Autodesk Fusion 360 part; units mm, degrees
(part 9 of 11)
  spline S49 degree 5 poles (-5.4732, -19.6968) (-5.4704, -19.6982) (-5.465, -19.7011) (-5.4568, -19.7055) (-5.4459, -19.7113) (-5.4323, -19.7184) (-5.4187, -19.7254) (-5.405, -19.7324) (-5.3914, -19.7394) (-5.3777, -19.7462) (-5.364, -19.753) (-5.3504, -19.7597) (-5.3367, -19.7663) (-5.323, -19.7729) (-5.3093, -19.7793) (-5.2955, -19.7857) (-5.2818, -19.7921) (-5.2681, -19.7983) (-5.2544, -19.8045) (-5.2406, -19.8106) (-5.2269, -19.8166) (-5.2131, -19.8226) (-5.1993, -19.8284) (-5.1855, -19.8342) (-5.1718, -19.8399) (-5.158, -19.8456) (-5.1442, -19.8511) (-5.1304, -19.8566) (-5.1166, -19.862) (-5.1028, -19.8673) (-5.089, -19.8725) (-5.0751, -19.8776) (-5.0613, -19.8827) (-5.0475, -19.8877) (-5.0337, -19.8925) (-5.0198, -19.8973) (-5.006, -19.902) (-4.9921, -19.9067) (-4.9783, -19.9112) (-4.9644, -19.9156) (-4.9506, -19.92) (-4.9367, -19.9242) (-4.9229, -19.9284) (-4.909, -19.9325) (-4.8951, -19.9364) (-4.8813, -19.9403) (-4.8674, -19.9441) (-4.8535, -19.9478) (-4.8397, -19.9514) (-4.8258, -19.9548) (-4.8119, -19.9582) (-4.7981, -19.9615) (-4.7842, -19.9646) (-4.7703, -19.9676) (-4.7565, -19.9705) (-4.7426, -19.9733) (-4.7288, -19.976) (-4.7149, -19.9786) (-4.701, -19.9811) (-4.6872, -19.9835) (-4.6733, -19.9857) (-4.6595, -19.9877) (-4.6457, -19.9895) (-4.6318, -19.9912) (-4.618, -19.9927) (-4.6042, -19.9941) (-4.5904, -19.9954) (-4.5766, -19.9965) (-4.5628, -19.9976) (-4.549, -19.9984) (-4.5353, -19.9988) (-4.5243, -19.9987) (-4.516, -19.9984) (-4.5106, -19.998) (-4.5078, -19.9978) knots -1 -1 -1 -1 -1 -1 -0.98571429 -0.97142857 -0.95714286 -0.94285714 -0.92857143 -0.91428571 -0.9 -0.88571429 -0.87142857 -0.85714286 -0.84285714 -0.82857143 -0.81428571 -0.8 -0.78571429 -0.77142857 -0.75714286 -0.74285714 -0.72857143 -0.71428571 -0.7 -0.68571429 -0.67142857 -0.65714286 -0.64285714 -0.62857143 -0.61428571 -0.6 -0.58571429 -0.57142857 -0.55714286 -0.54285714 -0.52857143 -0.51428571 -0.5 -0.48571429 -0.47142857 -0.45714286 -0.44285714 -0.42857143 -0.41428571 -0.4 -0.38571429 -0.37142857 -0.35714286 -0.34285714 -0.32857143 -0.31428571 -0.3 -0.28571429 -0.27142857 -0.25714286 -0.24285714 -0.22857143 -0.21428571 -0.2 -0.18571429 -0.17142857 -0.15714286 -0.14285714 -0.12857143 -0.11428571 -0.1 -0.08571429 -0.07142857 -0.05714286 -0.04285714 -0.02857143 -0.01428571 0 0 0 0 0 0
  line L57 (-4.5078, -19.9978) -> (-4.4395, -19.9925)
  arc A107 (-4.1719, -20.2115) -> (-4.4395, -19.9925) centre (-4.4201, -20.2417) ccw
  arc A108 (-4.1719, -20.2115) -> (-4.1569, -20.3258) centre (1.6741, -19.5) ccw
  arc A109 (-4.3587, -20.6066) -> (-4.1569, -20.3258) centre (-4.4044, -20.3608) ccw
  line L58 (-4.3587, -20.6066) -> (-4.426, -20.6192)
  spline S50 degree 5 poles (-4.426, -20.6192) (-4.4287, -20.6197) (-4.4341, -20.6207) (-4.4422, -20.6225) (-4.4528, -20.6253) (-4.466, -20.6293) (-4.4791, -20.6336) (-4.4921, -20.6382) (-4.5051, -20.6429) (-4.5181, -20.6477) (-4.5311, -20.6526) (-4.5441, -20.6577) (-4.557, -20.6628) (-4.5699, -20.6682) (-4.5828, -20.6737) (-4.5956, -20.6794) (-4.6083, -20.6853) (-4.6211, -20.6913) (-4.6338, -20.6974) (-4.6465, -20.7036) (-4.6591, -20.7099) (-4.6718, -20.7162) (-4.6844, -20.7228) (-4.697, -20.7294) (-4.7095, -20.7361) (-4.722, -20.743) (-4.7345, -20.7499) (-4.747, -20.757) (-4.7595, -20.7641) (-4.7719, -20.7713) (-4.7843, -20.7787) (-4.7966, -20.7861) (-4.809, -20.7936) (-4.8213, -20.8012) (-4.8335, -20.8089) (-4.8458, -20.8167) (-4.858, -20.8246) (-4.8702, -20.8325) (-4.8824, -20.8406) (-4.8946, -20.8487) (-4.9067, -20.8569) (-4.9188, -20.8652) (-4.9309, -20.8736) (-4.9429, -20.8821) (-4.9549, -20.8906) (-4.9669, -20.8992) (-4.9789, -20.9079) (-4.9908, -20.9167) (-5.0027, -20.9256) (-5.0146, -20.9345) (-5.0265, -20.9435) (-5.0383, -20.9526) (-5.0501, -20.9617) (-5.0619, -20.971) (-5.0737, -20.9803) (-5.0854, -20.9896) (-5.0971, -20.9991) (-5.1088, -21.0086) (-5.1204, -21.0182) (-5.132, -21.0279) (-5.1436, -21.0376) (-5.1552, -21.0474) (-5.1667, -21.0573) (-5.1782, -21.0672) (-5.1897, -21.0773) (-5.2012, -21.0873) (-5.2126, -21.0975) (-5.224, -21.1077) (-5.2353, -21.118) (-5.2467, -21.1283) (-5.258, -21.1388) (-5.267, -21.1471) (-5.2738, -21.1535) (-5.2783, -21.1577) (-5.2805, -21.1598) knots 0 0 0 0 0 0 0.01428571 0.02857143 0.04285714 0.05714286 0.07142857 0.08571429 0.1 0.11428571 0.12857143 0.14285714 0.15714286 0.17142857 0.18571429 0.2 0.21428571 0.22857143 0.24285714 0.25714286 0.27142857 0.28571429 0.3 0.31428571 0.32857143 0.34285714 0.35714286 0.37142857 0.38571429 0.4 0.41428571 0.42857143 0.44285714 0.45714286 0.47142857 0.48571429 0.5 0.51428571 0.52857143 0.54285714 0.55714286 0.57142857 0.58571429 0.6 0.61428571 0.62857143 0.64285714 0.65714286 0.67142857 0.68571429 0.7 0.71428571 0.72857143 0.74285714 0.75714286 0.77142857 0.78571429 0.8 0.81428571 0.82857143 0.84285714 0.85714286 0.87142857 0.88571429 0.9 0.91428571 0.92857143 0.94285714 0.95714286 0.97142857 0.98571429 1 1 1 1 1 1
  arc A110 (-5.2805, -21.1598) -> (-5.1787, -21.5399) centre (1.6741, -19.5) ccw
  spline S51 degree 5 poles (-5.1787, -21.5399) (-5.1757, -21.5406) (-5.1697, -21.542) (-5.1607, -21.5441) (-5.1486, -21.5469) (-5.1336, -21.5502) (-5.1186, -21.5535) (-5.1037, -21.5567) (-5.0887, -21.5599) (-5.0737, -21.563) (-5.0587, -21.566) (-5.0438, -21.5689) (-5.0289, -21.5718) (-5.0139, -21.5745) (-4.999, -21.5773) (-4.9841, -21.5799) (-4.9692, -21.5825) (-4.9543, -21.5849) (-4.9395, -21.5874) (-4.9246, -21.5897) (-4.9098, -21.5919) (-4.8949, -21.5941) (-4.8801, -21.5962) (-4.8653, -21.5983) (-4.8505, -21.6002) (-4.8357, -21.6021) (-4.821, -21.6039) (-4.8062, -21.6056) (-4.7915, -21.6072) (-4.7768, -21.6088) (-4.7621, -21.6102) (-4.7474, -21.6116) (-4.7328, -21.6129) (-4.7181, -21.6141) (-4.7035, -21.6153) (-4.6889, -21.6163) (-4.6743, -21.6173) (-4.6597, -21.6182) (-4.6452, -21.619) (-4.6306, -21.6197) (-4.6161, -21.6203) (-4.6017, -21.6208) (-4.5872, -21.6212) (-4.5728, -21.6216) (-4.5583, -21.6218) (-4.5439, -21.622) (-4.5296, -21.622) (-4.5152, -21.622) (-4.5009, -21.6219) (-4.4866, -21.6217) (-4.4723, -21.6213) (-4.4581, -21.6209) (-4.4439, -21.6203) (-4.4297, -21.6197) (-4.4156, -21.6189) (-4.4015, -21.618) (-4.3874, -21.617) (-4.3733, -21.6159) (-4.3593, -21.6147) (-4.3453, -21.6134) (-4.3314, -21.612) (-4.3175, -21.6103) (-4.3036, -21.6085) (-4.2898, -21.6066) (-4.2761, -21.6044) (-4.2624, -21.6022) (-4.2487, -21.5998) (-4.2351, -21.5974) (-4.2215, -21.5949) (-4.208, -21.5921) (-4.1946, -21.5889) (-4.184, -21.586) (-4.1761, -21.5835) (-4.1709, -21.5818) (-4.1683, -21.5809) knots -1 -1 -1 -1 -1 -1 -0.98571429 -0.97142857 -0.95714286 -0.94285714 -0.92857143 -0.91428571 -0.9 -0.88571429 -0.87142857 -0.85714286 -0.84285714 -0.82857143 -0.81428571 -0.8 -0.78571429 -0.77142857 -0.75714286 -0.74285714 -0.72857143 -0.71428571 -0.7 -0.68571429 -0.67142857 -0.65714286 -0.64285714 -0.62857143 -0.61428571 -0.6 -0.58571429 -0.57142857 -0.55714286 -0.54285714 -0.52857143 -0.51428571 -0.5 -0.48571429 -0.47142857 -0.45714286 -0.44285714 -0.42857143 -0.41428571 -0.4 -0.38571429 -0.37142857 -0.35714286 -0.34285714 -0.32857143 -0.31428571 -0.3 -0.28571429 -0.27142857 -0.25714286 -0.24285714 -0.22857143 -0.21428571 -0.2 -0.18571429 -0.17142857 -0.15714286 -0.14285714 -0.12857143 -0.11428571 -0.1 -0.08571429 -0.07142857 -0.05714286 -0.04285714 -0.02857143 -0.01428571 0 0 0 0 0 0
  line L59 (-4.1683, -21.5809) -> (-4.1038, -21.558)
  arc A111 (-3.7886, -21.7004) -> (-4.1038, -21.558) centre (-4.0205, -21.7938) ccw
  arc A112 (-3.7886, -21.7004) -> (-3.7445, -21.8068) centre (1.6741, -19.5) ccw
  arc A113 (-3.8667, -22.1303) -> (-3.7445, -21.8068) centre (-3.9745, -21.9048) ccw
  line L60 (-3.8667, -22.1303) -> (-3.9285, -22.1599)
  spline S52 degree 5 poles (-3.9285, -22.1599) (-3.931, -22.161) (-3.9359, -22.1635) (-3.9432, -22.1673) (-3.9528, -22.1727) (-3.9645, -22.18) (-3.976, -22.1875) (-3.9874, -22.1953) (-3.9988, -22.2033) (-4.0101, -22.2113) (-4.0214, -22.2194) (-4.0326, -22.2276) (-4.0437, -22.236) (-4.0548, -22.2445) (-4.0658, -22.2531) (-4.0767, -22.262) (-4.0875, -22.2709) (-4.0982, -22.28) (-4.109, -22.2892) (-4.1196, -22.2984) (-4.1302, -22.3078) (-4.1408, -22.3173) (-4.1513, -22.3268) (-4.1617, -22.3365) (-4.1721, -22.3462) (-4.1824, -22.3561) (-4.1927, -22.366) (-4.2029, -22.376) (-4.2131, -22.3862) (-4.2232, -22.3964) (-4.2332, -22.4067) (-4.2433, -22.417) (-4.2532, -22.4275) (-4.2632, -22.438) (-4.273, -22.4486) (-4.2828, -22.4593) (-4.2926, -22.4701) (-4.3023, -22.481) (-4.312, -22.4919) (-4.3217, -22.5029) (-4.3312, -22.5139) (-4.3408, -22.5251) (-4.3503, -22.5363) (-4.3597, -22.5476) (-4.3691, -22.559) (-4.3785, -22.5704) (-4.3878, -22.5819) (-4.397, -22.5935) (-4.4063, -22.6051) (-4.4154, -22.6168) (-4.4246, -22.6286) (-4.4336, -22.6404) (-4.4427, -22.6523) (-4.4517, -22.6643) (-4.4606, -22.6763) (-4.4695, -22.6884) (-4.4784, -22.7005) (-4.4872, -22.7128) (-4.4959, -22.725) (-4.5047, -22.7374) (-4.5133, -22.7498) (-4.522, -22.7623) (-4.5306, -22.7748) (-4.5391, -22.7874) (-4.5476, -22.8) (-4.556, -22.8127) (-4.5645, -22.8255) (-4.5728, -22.8383) (-4.5811, -22.8512) (-4.5894, -22.8641) (-4.5977, -22.8771) (-4.6042, -22.8875) (-4.6091, -22.8954) (-4.6123, -22.9006) (-4.614, -22.9033) knots 0 0 0 0 0 0 0.01428571 0.02857143 0.04285714 0.05714286 0.07142857 0.08571429 0.1 0.11428571 0.12857143 0.14285714 0.15714286 0.17142857 0.18571429 0.2 0.21428571 0.22857143 0.24285714 0.25714286 0.27142857 0.28571429 0.3 0.31428571 0.32857143 0.34285714 0.35714286 0.37142857 0.38571429 0.4 0.41428571 0.42857143 0.44285714 0.45714286 0.47142857 0.48571429 0.5 0.51428571 0.52857143 0.54285714 0.55714286 0.57142857 0.58571429 0.6 0.61428571 0.62857143 0.64285714 0.65714286 0.67142857 0.68571429 0.7 0.71428571 0.72857143 0.74285714 0.75714286 0.77142857 0.78571429 0.8 0.81428571 0.82857143 0.84285714 0.85714286 0.87142857 0.88571429 0.9 0.91428571 0.92857143 0.94285714 0.95714286 0.97142857 0.98571429 1 1 1 1 1 1
  arc A114 (-4.614, -22.9033) -> (-4.4172, -23.244) centre (1.6741, -19.5) ccw
  spline S53 degree 5 poles (-4.4172, -23.244) (-4.4141, -23.2439) (-4.408, -23.2438) (-4.3987, -23.2434) (-4.3864, -23.243) (-4.371, -23.2424) (-4.3557, -23.2417) (-4.3404, -23.2409) (-4.3251, -23.24) (-4.3098, -23.2391) (-4.2946, -23.2382) (-4.2794, -23.2371) (-4.2642, -23.236) (-4.2491, -23.2349) (-4.234, -23.2336) (-4.2189, -23.2323) (-4.2039, -23.2309) (-4.1888, -23.2295) (-4.1739, -23.228) (-4.1589, -23.2264) (-4.144, -23.2247) (-4.1291, -23.223) (-4.1142, -23.2212) (-4.0994, -23.2193) (-4.0846, -23.2173) (-4.0699, -23.2153) (-4.0551, -23.2132) (-4.0405, -23.2111) (-4.0258, -23.2088) (-4.0112, -23.2065) (-3.9966, -23.2041) (-3.9821, -23.2017) (-3.9676, -23.1991) (-3.9531, -23.1965) (-3.9387, -23.1938) (-3.9243, -23.1911) (-3.91, -23.1882) (-3.8957, -23.1853) (-3.8814, -23.1823) (-3.8672, -23.1792) (-3.853, -23.1761) (-3.8389, -23.1728) (-3.8248, -23.1695) (-3.8108, -23.1661) (-3.7968, -23.1626) (-3.7829, -23.159) (-3.769, -23.1554) (-3.7551, -23.1516) (-3.7413, -23.1478) (-3.7276, -23.1439) (-3.7139, -23.1399) (-3.7002, -23.1358) (-3.6866, -23.1315) (-3.6731, -23.1272) (-3.6597, -23.1228) (-3.6463, -23.1183) (-3.6329, -23.1137) (-3.6196, -23.109) (-3.6064, -23.1043) (-3.5932, -23.0994) (-3.5801, -23.0943) (-3.5671, -23.0892) (-3.5542, -23.0838) (-3.5414, -23.0784) (-3.5287, -23.0728) (-3.516, -23.067) (-3.5034, -23.0612) (-3.4909, -23.0554) (-3.4784, -23.0494) (-3.4661, -23.0432) (-3.454, -23.0367) (-3.4445, -23.0311) (-3.4375, -23.0267) (-3.433, -23.0237) (-3.4307, -23.0221) knots -1 -1 -1 -1 -1 -1 -0.98571429 -0.97142857 -0.95714286 -0.94285714 -0.92857143 -0.91428571 -0.9 -0.88571429 -0.87142857 -0.85714286 -0.84285714 -0.82857143 -0.81428571 -0.8 -0.78571429 -0.77142857 -0.75714286 -0.74285714 -0.72857143 -0.71428571 -0.7 -0.68571429 -0.67142857 -0.65714286 -0.64285714 -0.62857143 -0.61428571 -0.6 -0.58571429 -0.57142857 -0.55714286 -0.54285714 -0.52857143 -0.51428571 -0.5 -0.48571429 -0.47142857 -0.45714286 -0.44285714 -0.42857143 -0.41428571 -0.4 -0.38571429 -0.37142857 -0.35714286 -0.34285714 -0.32857143 -0.31428571 -0.3 -0.28571429 -0.27142857 -0.25714286 -0.24285714 -0.22857143 -0.21428571 -0.2 -0.18571429 -0.17142857 -0.15714286 -0.14285714 -0.12857143 -0.11428571 -0.1 -0.08571429 -0.07142857 -0.05714286 -0.04285714 -0.02857143 -0.01428571 0 0 0 0 0 0
  line L61 (-3.4307, -23.0221) -> (-3.3742, -22.9833)
  arc A115 (-3.0329, -23.0392) -> (-3.3742, -22.9833) centre (-3.2328, -23.1895) ccw
  arc A116 (-3.0329, -23.0392) -> (-2.9628, -23.1307) centre (1.6741, -19.5) ccw
  arc A117 (-2.9971, -23.4748) -> (-2.9628, -23.1307) centre (-3.1596, -23.2848) ccw
  line L62 (-2.9971, -23.4748) -> (-3.0492, -23.5193)
  spline S54 degree 5 poles (-3.0492, -23.5193) (-3.0513, -23.5211) (-3.0554, -23.5247) (-3.0615, -23.5303) (-3.0693, -23.538) (-3.0787, -23.548) (-3.0879, -23.5583) (-3.0969, -23.5688) (-3.1058, -23.5794) (-3.1147, -23.5901) (-3.1235, -23.6008) (-3.1322, -23.6117) (-3.1408, -23.6226) (-3.1493, -23.6337) (-3.1576, -23.6449) (-3.1659, -23.6563) (-3.174, -23.6677) (-3.182, -23.6793) (-3.19, -23.6909) (-3.1979, -23.7026) (-3.2057, -23.7144) (-3.2135, -23.7263) (-3.2211, -23.7382) (-3.2287, -23.7502) (-3.2362, -23.7623) (-3.2436, -23.7745) (-3.251, -23.7868) (-3.2583, -23.7991) (-3.2655, -23.8115) (-3.2726, -23.824) (-3.2797, -23.8366) (-3.2866, -23.8492) (-3.2936, -23.8619) (-3.3004, -23.8746) (-3.3072, -23.8874) (-3.3139, -23.9003) (-3.3206, -23.9132) (-3.3272, -23.9262) (-3.3337, -23.9393) (-3.3402, -23.9524) (-3.3466, -23.9656) (-3.3529, -23.9788) (-3.3591, -23.9921) (-3.3653, -24.0054) (-3.3715, -24.0188) (-3.3776, -24.0323) (-3.3836, -24.0458) (-3.3895, -24.0594) (-3.3954, -24.073) (-3.4012, -24.0867) (-3.407, -24.1004) (-3.4127, -24.1142) (-3.4184, -24.128) (-3.424, -24.1419) (-3.4295, -24.1558) (-3.435, -24.1698) (-3.4404, -24.1839) (-3.4457, -24.198) (-3.451, -24.2121) (-3.4562, -24.2263) (-3.4614, -24.2405) (-3.4665, -24.2548) (-3.4716, -24.2691) (-3.4766, -24.2834) (-3.4815, -24.2979) (-3.4864, -24.3123) (-3.4912, -24.3268) (-3.496, -24.3414) (-3.5007, -24.356) (-3.5053, -24.3706) (-3.5099, -24.3853) (-3.5135, -24.3971) (-3.5162, -24.4059) (-3.518, -24.4118) (-3.5189, -24.4148) knots 0 0 0 0 0 0 0.01428571 0.02857143 0.04285714 0.05714286 0.07142857 0.08571429 0.1 0.11428571 0.12857143 0.14285714 0.15714286 0.17142857 0.18571429 0.2 0.21428571 0.22857143 0.24285714 0.25714286 0.27142857 0.28571429 0.3 0.31428571 0.32857143 0.34285714 0.35714286 0.37142857 0.38571429 0.4 0.41428571 0.42857143 0.44285714 0.45714286 0.47142857 0.48571429 0.5 0.51428571 0.52857143 0.54285714 0.55714286 0.57142857 0.58571429 0.6 0.61428571 0.62857143 0.64285714 0.65714286 0.67142857 0.68571429 0.7 0.71428571 0.72857143 0.74285714 0.75714286 0.77142857 0.78571429 0.8 0.81428571 0.82857143 0.84285714 0.85714286 0.87142857 0.88571429 0.9 0.91428571 0.92857143 0.94285714 0.95714286 0.97142857 0.98571429 1 1 1 1 1 1
  arc A118 (-3.5189, -24.4148) -> (-3.2406, -24.693) centre (1.6741, -19.5) ccw
  spline S55 degree 5 poles (-3.2406, -24.693) (-3.2377, -24.6921) (-3.2318, -24.6904) (-3.2229, -24.6877) (-3.2111, -24.684) (-3.1965, -24.6794) (-3.1818, -24.6748) (-3.1672, -24.6701) (-3.1527, -24.6653) (-3.1382, -24.6605) (-3.1237, -24.6556) (-3.1093, -24.6507) (-3.0949, -24.6457) (-3.0806, -24.6406) (-3.0663, -24.6355) (-3.0521, -24.6304) (-3.0379, -24.6251) (-3.0238, -24.6198) (-3.0097, -24.6145) (-2.9957, -24.6091) (-2.9817, -24.6036) (-2.9678, -24.5981) (-2.9539, -24.5925) (-2.9401, -24.5869) (-2.9263, -24.5812) (-2.9125, -24.5754) (-2.8989, -24.5696) (-2.8852, -24.5637) (-2.8717, -24.5577) (-2.8582, -24.5517) (-2.8447, -24.5456) (-2.8313, -24.5395) (-2.8179, -24.5333) (-2.8047, -24.527) (-2.7914, -24.5207) (-2.7782, -24.5143) (-2.7651, -24.5078) (-2.7521, -24.5013) (-2.7391, -24.4947) (-2.7261, -24.4881) (-2.7133, -24.4814) (-2.7005, -24.4746) (-2.6877, -24.4677) (-2.675, -24.4608) (-2.6624, -24.4538) (-2.6499, -24.4467) (-2.6374, -24.4396) (-2.625, -24.4324) (-2.6127, -24.4251) (-2.6004, -24.4178) (-2.5882, -24.4104) (-2.5761, -24.4029) (-2.5641, -24.3953) (-2.5521, -24.3876) (-2.5403, -24.3799) (-2.5285, -24.372) (-2.5168, -24.3641) (-2.5051, -24.3562) (-2.4936, -24.3481) (-2.4821, -24.34) (-2.4708, -24.3318) (-2.4596, -24.3234) (-2.4485, -24.3149) (-2.4375, -24.3063) (-2.4267, -24.2976) (-2.416, -24.2888) (-2.4053, -24.2799) (-2.3947, -24.271) (-2.3842, -24.262) (-2.3739, -24.2529) (-2.3639, -24.2434) (-2.3561, -24.2356) (-2.3506, -24.2295) (-2.3469, -24.2254) (-2.3452, -24.2233) knots -1 -1 -1 -1 -1 -1 -0.98571429 -0.97142857 -0.95714286 -0.94285714 -0.92857143 -0.91428571 -0.9 -0.88571429 -0.87142857 -0.85714286 -0.84285714 -0.82857143 -0.81428571 -0.8 -0.78571429 -0.77142857 -0.75714286 -0.74285714 -0.72857143 -0.71428571 -0.7 -0.68571429 -0.67142857 -0.65714286 -0.64285714 -0.62857143 -0.61428571 -0.6 -0.58571429 -0.57142857 -0.55714286 -0.54285714 -0.52857143 -0.51428571 -0.5 -0.48571429 -0.47142857 -0.45714286 -0.44285714 -0.42857143 -0.41428571 -0.4 -0.38571429 -0.37142857 -0.35714286 -0.34285714 -0.32857143 -0.31428571 -0.3 -0.28571429 -0.27142857 -0.25714286 -0.24285714 -0.22857143 -0.21428571 -0.2 -0.18571429 -0.17142857 -0.15714286 -0.14285714 -0.12857143 -0.11428571 -0.1 -0.08571429 -0.07142857 -0.05714286 -0.04285714 -0.02857143 -0.01428571 0 0 0 0 0 0
  line L63 (-2.3452, -24.2233) -> (-2.3006, -24.1713)
  arc A119 (-1.9565, -24.1369) -> (-2.3006, -24.1713) centre (-2.1106, -24.3338) ccw
  arc A120 (-1.9565, -24.1369) -> (-1.8651, -24.2071) centre (1.6741, -19.5) ccw
  arc A121 (-1.8092, -24.5484) -> (-1.8651, -24.2071) centre (-2.0153, -24.4069) ccw
  line L64 (-1.8092, -24.5484) -> (-1.848, -24.6048)
  spline S56 degree 5 poles (-1.848, -24.6048) (-1.8495, -24.6071) (-1.8526, -24.6117) (-1.857, -24.6186) (-1.8626, -24.6281) (-1.8691, -24.6402) (-1.8753, -24.6525) (-1.8812, -24.665) (-1.8871, -24.6776) (-1.8929, -24.6902) (-1.8986, -24.7028) (-1.9042, -24.7155) (-1.9097, -24.7283) (-1.915, -24.7412) (-1.9202, -24.7542) (-1.9252, -24.7673) (-1.9301, -24.7805) (-1.9349, -24.7937) (-1.9396, -24.807) (-1.9442, -24.8204) (-1.9487, -24.8338) (-1.9531, -24.8473) (-1.9574, -24.8608) (-1.9616, -24.8744) (-1.9657, -24.888) (-1.9697, -24.9017) (-1.9737, -24.9154) (-1.9775, -24.9292) (-1.9812, -24.9431) (-1.9849, -24.957) (-1.9885, -24.9709) (-1.992, -24.9849) (-1.9954, -24.999) (-1.9987, -25.013) (-2.0019, -25.0272) (-2.0051, -25.0413) (-2.0082, -25.0556) (-2.0112, -25.0698) (-2.0141, -25.0841) (-2.0169, -25.0985) (-2.0197, -25.1128) (-2.0224, -25.1273) (-2.025, -25.1417) (-2.0275, -25.1562) (-2.03, -25.1708) (-2.0324, -25.1853) (-2.0347, -25.2) (-2.0369, -25.2146) (-2.0391, -25.2293) (-2.0412, -25.244) (-2.0432, -25.2588) (-2.0452, -25.2735) (-2.047, -25.2884) (-2.0488, -25.3032) (-2.0506, -25.3181) (-2.0522, -25.333) (-2.0538, -25.348) (-2.0553, -25.363) (-2.0568, -25.378) (-2.0582, -25.3931) (-2.0595, -25.4081) (-2.0607, -25.4232) (-2.0619, -25.4384) (-2.063, -25.4536) (-2.064, -25.4688) (-2.065, -25.484) (-2.0659, -25.4992) (-2.0667, -25.5145) (-2.0675, -25.5298) (-2.0682, -25.5452) (-2.0688, -25.5605) (-2.0693, -25.5729) (-2.0696, -25.5821) (-2.0698, -25.5883) (-2.0699, -25.5914) knots 0 0 0 0 0 0 0.01428571 0.02857143 0.04285714 0.05714286 0.07142857 0.08571429 0.1 0.11428571 0.12857143 0.14285714 0.15714286 0.17142857 0.18571429 0.2 0.21428571 0.22857143 0.24285714 0.25714286 0.27142857 0.28571429 0.3 0.31428571 0.32857143 0.34285714 0.35714286 0.37142857 0.38571429 0.4 0.41428571 0.42857143 0.44285714 0.45714286 0.47142857 0.48571429 0.5 0.51428571 0.52857143 0.54285714 0.55714286 0.57142857 0.58571429 0.6 0.61428571 0.62857143 0.64285714 0.65714286 0.67142857 0.68571429 0.7 0.71428571 0.72857143 0.74285714 0.75714286 0.77142857 0.78571429 0.8 0.81428571 0.82857143 0.84285714 0.85714286 0.87142857 0.88571429 0.9 0.91428571 0.92857143 0.94285714 0.95714286 0.97142857 0.98571429 1 1 1 1 1 1
  arc A122 (-2.0699, -25.5914) -> (-1.7291, -25.7881) centre (1.6741, -19.5) ccw
  spline S57 degree 5 poles (-1.7291, -25.7881) (-1.7265, -25.7865) (-1.7212, -25.7832) (-1.7134, -25.7783) (-1.7029, -25.7718) (-1.69, -25.7636) (-1.677, -25.7553) (-1.6641, -25.747) (-1.6513, -25.7386) (-1.6386, -25.7302) (-1.6259, -25.7217) (-1.6132, -25.7132) (-1.6006, -25.7047) (-1.5881, -25.6961) (-1.5756, -25.6875) (-1.5632, -25.6788) (-1.5509, -25.6701) (-1.5386, -25.6613) (-1.5264, -25.6525) (-1.5142, -25.6436) (-1.5022, -25.6347) (-1.4901, -25.6258) (-1.4782, -25.6168) (-1.4663, -25.6078) (-1.4544, -25.5987) (-1.4427, -25.5896) (-1.431, -25.5804) (-1.4193, -25.5712) (-1.4077, -25.5619) (-1.3962, -25.5526) (-1.3848, -25.5433) (-1.3735, -25.5339) (-1.3622, -25.5244) (-1.351, -25.5149) (-1.3398, -25.5054) (-1.3287, -25.4958) (-1.3177, -25.4862) (-1.3068, -25.4765) (-1.296, -25.4668) (-1.2852, -25.457) (-1.2745, -25.4472) (-1.2639, -25.4373) (-1.2533, -25.4274) (-1.2429, -25.4174) (-1.2325, -25.4074) (-1.2222, -25.3973) (-1.212, -25.3872) (-1.2019, -25.377) (-1.1919, -25.3668) (-1.1819, -25.3565) (-1.1721, -25.3462) (-1.1623, -25.3358) (-1.1527, -25.3254) (-1.1431, -25.3149) (-1.1337, -25.3044) (-1.1243, -25.2937) (-1.115, -25.2831) (-1.1059, -25.2724) (-1.0968, -25.2616) (-1.0878, -25.2508) (-1.079, -25.2399) (-1.0703, -25.2289) (-1.0618, -25.2179) (-1.0535, -25.2067) (-1.0453, -25.1955) (-1.0372, -25.1842) (-1.0291, -25.1729) (-1.0212, -25.1616) (-1.0134, -25.1501) (-1.0058, -25.1386) (-0.9986, -25.1269) (-0.9931, -25.1174) (-0.9893, -25.1101) (-0.9869, -25.1051) (-0.9857, -25.1026) knots -1 -1 -1 -1 -1 -1 -0.98571429 -0.97142857 -0.95714286 -0.94285714 -0.92857143 -0.91428571 -0.9 -0.88571429 -0.87142857 -0.85714286 -0.84285714 -0.82857143 -0.81428571 -0.8 -0.78571429 -0.77142857 -0.75714286 -0.74285714 -0.72857143 -0.71428571 -0.7 -0.68571429 -0.67142857 -0.65714286 -0.64285714 -0.62857143 -0.61428571 -0.6 -0.58571429 -0.57142857 -0.55714286 -0.54285714 -0.52857143 -0.51428571 -0.5 -0.48571429 -0.47142857 -0.45714286 -0.44285714 -0.42857143 -0.41428571 -0.4 -0.38571429 -0.37142857 -0.35714286 -0.34285714 -0.32857143 -0.31428571 -0.3 -0.28571429 -0.27142857 -0.25714286 -0.24285714 -0.22857143 -0.21428571 -0.2 -0.18571429 -0.17142857 -0.15714286 -0.14285714 -0.12857143 -0.11428571 -0.1 -0.08571429 -0.07142857 -0.05714286 -0.04285714 -0.02857143 -0.01428571 0 0 0 0 0 0
  line L65 (-0.9857, -25.1026) -> (-0.9562, -25.0408)
  arc A123 (-0.6327, -24.9186) -> (-0.9562, -25.0408) centre (-0.7306, -25.1486) ccw
  arc A124 (-0.6327, -24.9186) -> (-0.5262, -24.9627) centre (1.6741, -19.5) ccw
  arc A125 (-0.3839, -25.2779) -> (-0.5262, -24.9627) centre (-0.6196, -25.1946) ccw
  line L66 (-0.3839, -25.2779) -> (-0.4067, -25.3425)
  spline S58 degree 5 poles (-0.4067, -25.3425) (-0.4076, -25.3451) (-0.4094, -25.3503) (-0.4119, -25.3581) (-0.4148, -25.3687) (-0.4179, -25.3821) (-0.4207, -25.3956) (-0.4233, -25.4092) (-0.4257, -25.4229) (-0.428, -25.4365) (-0.4303, -25.4502) (-0.4324, -25.464) (-0.4344, -25.4778) (-0.4362, -25.4916) (-0.4378, -25.5055) (-0.4393, -25.5194) (-0.4406, -25.5334) (-0.4418, -25.5475) (-0.4429, -25.5615) (-0.4439, -25.5756) (-0.4447, -25.5897) (-0.4455, -25.6039) (-0.4462, -25.618) (-0.4467, -25.6322) (-0.4472, -25.6465) (-0.4475, -25.6607) (-0.4477, -25.675) (-0.4479, -25.6894) (-0.4479, -25.7037) (-0.4478, -25.7181) (-0.4477, -25.7325) (-0.4474, -25.7469) (-0.4471, -25.7613) (-0.4467, -25.7758) (-0.4461, -25.7903) (-0.4455, -25.8048) (-0.4448, -25.8193) (-0.444, -25.8339) (-0.4431, -25.8484) (-0.4422, -25.863) (-0.4411, -25.8776) (-0.44, -25.8923) (-0.4388, -25.9069) (-0.4375, -25.9216) (-0.4361, -25.9362) (-0.4346, -25.9509) (-0.4331, -25.9656) (-0.4314, -25.9804) (-0.4297, -25.9951) (-0.4279, -26.0099) (-0.4261, -26.0247) (-0.4241, -26.0394) (-0.4221, -26.0542) (-0.42, -26.0691) (-0.4178, -26.0839) (-0.4155, -26.0987) (-0.4132, -26.1136) (-0.4108, -26.1285) (-0.4083, -26.1433) (-0.4058, -26.1582) (-0.4031, -26.1731) (-0.4004, -26.1881) (-0.3976, -26.203) (-0.3948, -26.2179) (-0.3918, -26.2329) (-0.3888, -26.2478) (-0.3858, -26.2628) (-0.3826, -26.2778) (-0.3794, -26.2928) (-0.3761, -26.3078) (-0.3727, -26.3228) (-0.37, -26.3348) (-0.3679, -26.3438) (-0.3665, -26.3498) (-0.3658, -26.3528) knots 0 0 0 0 0 0 0.01428571 0.02857143 0.04285714 0.05714286 0.07142857 0.08571429 0.1 0.11428571 0.12857143 0.14285714 0.15714286 0.17142857 0.18571429 0.2 0.21428571 0.22857143 0.24285714 0.25714286 0.27142857 0.28571429 0.3 0.31428571 0.32857143 0.34285714 0.35714286 0.37142857 0.38571429 0.4 0.41428571 0.42857143 0.44285714 0.45714286 0.47142857 0.48571429 0.5 0.51428571 0.52857143 0.54285714 0.55714286 0.57142857 0.58571429 0.6 0.61428571 0.62857143 0.64285714 0.65714286 0.67142857 0.68571429 0.7 0.71428571 0.72857143 0.74285714 0.75714286 0.77142857 0.78571429 0.8 0.81428571 0.82857143 0.84285714 0.85714286 0.87142857 0.88571429 0.9 0.91428571 0.92857143 0.94285714 0.95714286 0.97142857 0.98571429 1 1 1 1 1 1
  arc A126 (-0.3658, -26.3528) -> (0.0143, -26.4547) centre (1.6741, -19.5) ccw
  spline S59 degree 5 poles (0.0143, -26.4547) (0.0164, -26.4524) (0.0207, -26.4479) (0.027, -26.4412) (0.0354, -26.4321) (0.0458, -26.4208) (0.0562, -26.4095) (0.0664, -26.3981) (0.0767, -26.3867) (0.0868, -26.3753) (0.0969, -26.3638) (0.1069, -26.3524) (0.1168, -26.3408) (0.1267, -26.3293) (0.1365, -26.3177) (0.1463, -26.3062) (0.1559, -26.2945) (0.1655, -26.2829) (0.175, -26.2712) (0.1845, -26.2595) (0.1939, -26.2478) (0.2032, -26.236) (0.2124, -26.2243) (0.2216, -26.2125) (0.2306, -26.2006) (0.2396, -26.1888) (0.2486, -26.1769) (0.2574, -26.165) (0.2662, -26.153) (0.2749, -26.1411) (0.2835, -26.1291) (0.2921, -26.117) (0.3005, -26.105) (0.3089, -26.0929) (0.3172, -26.0808) (0.3254, -26.0687) (0.3335, -26.0565) (0.3416, -26.0444) (0.3496, -26.0322) (0.3574, -26.0199) (0.3652, -26.0077) (0.3729, -25.9954) (0.3805, -25.9831) (0.388, -25.9708) (0.3955, -25.9584) (0.4028, -25.946) (0.41, -25.9336) (0.4172, -25.9211) (0.4242, -25.9087) (0.4312, -25.8962) (0.438, -25.8837) (0.4448, -25.8711) (0.4514, -25.8585) (0.4579, -25.8459) (0.4643, -25.8333) (0.4706, -25.8206) (0.4768, -25.8079) (0.4829, -25.7952) (0.4888, -25.7825) (0.4947, -25.7697) (0.5004, -25.7569) (0.5059, -25.7441) (0.5113, -25.7312) (0.5165, -25.7182) (0.5215, -25.7053) (0.5264, -25.6923) (0.5312, -25.6793) (0.536, -25.6662) (0.5405, -25.6532) (0.5449, -25.6401) (0.5488, -25.6269) (0.5516, -25.6163) (0.5534, -25.6083) (0.5545, -25.6029) (0.555, -25.6002) knots -1 -1 -1 -1 -1 -1 -0.98571429 -0.97142857 -0.95714286 -0.94285714 -0.92857143 -0.91428571 -0.9 -0.88571429 -0.87142857 -0.85714286 -0.84285714 -0.82857143 -0.81428571 -0.8 -0.78571429 -0.77142857 -0.75714286 -0.74285714 -0.72857143 -0.71428571 -0.7 -0.68571429 -0.67142857 -0.65714286 -0.64285714 -0.62857143 -0.61428571 -0.6 -0.58571429 -0.57142857 -0.55714286 -0.54285714 -0.52857143 -0.51428571 -0.5 -0.48571429 -0.47142857 -0.45714286 -0.44285714 -0.42857143 -0.41428571 -0.4 -0.38571429 -0.37142857 -0.35714286 -0.34285714 -0.32857143 -0.31428571 -0.3 -0.28571429 -0.27142857 -0.25714286 -0.24285714 -0.22857143 -0.21428571 -0.2 -0.18571429 -0.17142857 -0.15714286 -0.14285714 -0.12857143 -0.11428571 -0.1 -0.08571429 -0.07142857 -0.05714286 -0.04285714 -0.02857143 -0.01428571 0 0 0 0 0 0
  line L67 (0.555, -25.6002) -> (0.5675, -25.5328)
  arc A127 (0.8484, -25.331) -> (0.5675, -25.5328) centre (0.8133, -25.5785) ccw
  arc A128 (0.8484, -25.331) -> (0.9626, -25.3461) centre (1.6741, -19.5) ccw
  arc A129 (1.1816, -25.6137) -> (0.9626, -25.3461) centre (0.9324, -25.5942) ccw
  line L68 (1.1816, -25.6137) -> (1.1763, -25.682)
  spline S60 degree 5 poles (1.1763, -25.682) (1.1761, -25.6847) (1.1757, -25.6902) (1.1754, -25.6984) (1.1753, -25.7094) (1.1757, -25.7232) (1.1765, -25.7369) (1.1776, -25.7507) (1.1788, -25.7645) (1.1801, -25.7783) (1.1815, -25.7921) (1.183, -25.806) (1.1846, -25.8198) (1.1864, -25.8336) (1.1885, -25.8475) (1.1907, -25.8613) (1.193, -25.8752) (1.1955, -25.889) (1.1981, -25.9029) (1.2008, -25.9168) (1.2036, -25.9306) (1.2065, -25.9445) (1.2095, -25.9583) (1.2127, -25.9722) (1.2159, -25.9861) (1.2193, -25.9999) (1.2228, -26.0138) (1.2264, -26.0277) (1.23, -26.0415) (1.2338, -26.0554) (1.2377, -26.0693) (1.2417, -26.0831) (1.2457, -26.097) (1.2499, -26.1109) (1.2541, -26.1247) (1.2585, -26.1386) (1.2629, -26.1524) (1.2675, -26.1663) (1.2721, -26.1801) (1.2768, -26.194) (1.2816, -26.2078) (1.2865, -26.2216) (1.2915, -26.2355) (1.2965, -26.2493) (1.3016, -26.2631) (1.3069, -26.2769) (1.3122, -26.2907) (1.3176, -26.3045) (1.323, -26.3183) (1.3286, -26.3321) (1.3342, -26.3459) (1.3399, -26.3597) (1.3457, -26.3735) (1.3516, -26.3872) (1.3575, -26.401) (1.3635, -26.4147) (1.3696, -26.4285) (1.3758, -26.4422) (1.3821, -26.456) (1.3884, -26.4697) (1.3948, -26.4834) (1.4013, -26.4971) (1.4078, -26.5108) (1.4145, -26.5245) (1.4212, -26.5382) (1.4279, -26.5519) (1.4348, -26.5655) (1.4417, -26.5792) (1.4487, -26.5928) (1.4558, -26.6065) (1.4629, -26.6201) (1.4687, -26.631) (1.473, -26.6391) (1.4759, -26.6446) (1.4774, -26.6473) knots 0 0 0 0 0 0 0.01428571 0.02857143 0.04285714 0.05714286 0.07142857 0.08571429 0.1 0.11428571 0.12857143 0.14285714 0.15714286 0.17142857 0.18571429 0.2 0.21428571 0.22857143 0.24285714 0.25714286 0.27142857 0.28571429 0.3 0.31428571 0.32857143 0.34285714 0.35714286 0.37142857 0.38571429 0.4 0.41428571 0.42857143 0.44285714 0.45714286 0.47142857 0.48571429 0.5 0.51428571 0.52857143 0.54285714 0.55714286 0.57142857 0.58571429 0.6 0.61428571 0.62857143 0.64285714 0.65714286 0.67142857 0.68571429 0.7 0.71428571 0.72857143 0.74285714 0.75714286 0.77142857 0.78571429 0.8 0.81428571 0.82857143 0.84285714 0.85714286 0.87142857 0.88571429 0.9 0.91428571 0.92857143 0.94285714 0.95714286 0.97142857 0.98571429 1 1 1 1 1 1
  arc A130 (1.4774, -26.6473) -> (1.8709, -26.6473) centre (1.6741, -19.5) ccw
  spline S61 degree 5 poles (1.8709, -26.6473) (1.8724, -26.6446) (1.8753, -26.6391) (1.8796, -26.631) (1.8854, -26.6201) (1.8925, -26.6065) (1.8996, -26.5928) (1.9066, -26.5792) (1.9135, -26.5655) (1.9203, -26.5519) (1.9271, -26.5382) (1.9338, -26.5245) (1.9404, -26.5108) (1.947, -26.4971) (1.9535, -26.4834) (1.9599, -26.4697) (1.9662, -26.456) (1.9725, -26.4422) (1.9786, -26.4285) (1.9847, -26.4147) (1.9908, -26.401) (1.9967, -26.3872) (2.0026, -26.3735) (2.0084, -26.3597) (2.0141, -26.3459) (2.0197, -26.3321) (2.0253, -26.3183) (2.0307, -26.3045) (2.0361, -26.2907) (2.0414, -26.2769) (2.0466, -26.2631) (2.0518, -26.2493) (2.0568, -26.2355) (2.0618, -26.2216) (2.0667, -26.2078) (2.0715, -26.194) (2.0762, -26.1801) (2.0808, -26.1663) (2.0853, -26.1524) (2.0898, -26.1386) (2.0941, -26.1247) (2.0984, -26.1109) (2.1025, -26.097) (2.1066, -26.0831) (2.1106, -26.0693) (2.1145, -26.0554) (2.1182, -26.0415) (2.1219, -26.0277) (2.1255, -26.0138) (2.129, -25.9999) (2.1324, -25.9861) (2.1356, -25.9722) (2.1388, -25.9583) (2.1418, -25.9445) (2.1447, -25.9306) (2.1475, -25.9168) (2.1502, -25.9029) (2.1528, -25.889) (2.1553, -25.8752) (2.1576, -25.8613) (2.1598, -25.8475) (2.1618, -25.8336) (2.1637, -25.8198) (2.1653, -25.806) (2.1668, -25.7921) (2.1682, -25.7783) (2.1695, -25.7645) (2.1707, -25.7507) (2.1717, -25.7369) (2.1725, -25.7232) (2.173, -25.7094) (2.1729, -25.6984) (2.1725, -25.6902) (2.1722, -25.6847) (2.172, -25.682) knots -1 -1 -1 -1 -1 -1 -0.98571429 -0.97142857 -0.95714286 -0.94285714 -0.92857143 -0.91428571 -0.9 -0.88571429 -0.87142857 -0.85714286 -0.84285714 -0.82857143 -0.81428571 -0.8 -0.78571429 -0.77142857 -0.75714286 -0.74285714 -0.72857143 -0.71428571 -0.7 -0.68571429 -0.67142857 -0.65714286 -0.64285714 -0.62857143 -0.61428571 -0.6 -0.58571429 -0.57142857 -0.55714286 -0.54285714 -0.52857143 -0.51428571 -0.5 -0.48571429 -0.47142857 -0.45714286 -0.44285714 -0.42857143 -0.41428571 -0.4 -0.38571429 -0.37142857 -0.35714286 -0.34285714 -0.32857143 -0.31428571 -0.3 -0.28571429 -0.27142857 -0.25714286 -0.24285714 -0.22857143 -0.21428571 -0.2 -0.18571429 -0.17142857 -0.15714286 -0.14285714 -0.12857143 -0.11428571 -0.1 -0.08571429 -0.07142857 -0.05714286 -0.04285714 -0.02857143 -0.01428571 0 0 0 0 0 0
  line L69 (2.172, -25.682) -> (2.1666, -25.6137)
  arc A131 (2.3857, -25.3461) -> (2.1666, -25.6137) centre (2.4159, -25.5942) ccw
  arc A132 (2.3857, -25.3461) -> (2.4999, -25.331) centre (1.6741, -19.5) ccw
  arc A133 (2.7808, -25.5328) -> (2.4999, -25.331) centre (2.535, -25.5785) ccw
  line L70 (2.7808, -25.5328) -> (2.7933, -25.6002)
  spline S62 degree 5 poles (2.7933, -25.6002) (2.7938, -25.6029) (2.7949, -25.6083) (2.7967, -25.6163) (2.7994, -25.6269) (2.8034, -25.6401) (2.8077, -25.6532) (2.8123, -25.6662) (2.817, -25.6793) (2.8219, -25.6923) (2.8268, -25.7053) (2.8318, -25.7182) (2.837, -25.7312) (2.8423, -25.7441) (2.8479, -25.7569) (2.8536, -25.7697) (2.8594, -25.7825) (2.8654, -25.7952) (2.8715, -25.8079) (2.8777, -25.8206) (2.884, -25.8333) (2.8904, -25.8459) (2.8969, -25.8585) (2.9035, -25.8711) (2.9103, -25.8837) (2.9171, -25.8962) (2.9241, -25.9087) (2.9311, -25.9211) (2.9382, -25.9336) (2.9455, -25.946) (2.9528, -25.9584) (2.9602, -25.9708) (2.9678, -25.9831) (2.9754, -25.9954) (2.9831, -26.0077) (2.9908, -26.0199) (2.9987, -26.0322) (3.0067, -26.0444) (3.0147, -26.0565) (3.0229, -26.0687) (3.0311, -26.0808) (3.0394, -26.0929) (3.0478, -26.105) (3.0562, -26.117) (3.0648, -26.1291) (3.0734, -26.1411) (3.0821, -26.153) (3.0908, -26.165) (3.0997, -26.1769) (3.1086, -26.1888) (3.1176, -26.2006) (3.1267, -26.2125) (3.1359, -26.2243) (3.1451, -26.236) (3.1544, -26.2478) (3.1638, -26.2595) (3.1732, -26.2712) (3.1828, -26.2829) (3.1924, -26.2945) (3.202, -26.3062) (3.2118, -26.3177) (3.2216, -26.3293) (3.2314, -26.3408) (3.2414, -26.3524) (3.2514, -26.3638) (3.2615, -26.3753) (3.2716, -26.3867) (3.2818, -26.3981) (3.2921, -26.4095) (3.3025, -26.4208) (3.3129, -26.4321) (3.3213, -26.4412) (3.3276, -26.4479) (3.3318, -26.4524) (3.3339, -26.4547) knots 0 0 0 0 0 0 0.01428571 0.02857143 0.04285714 0.05714286 0.07142857 0.08571429 0.1 0.11428571 0.12857143 0.14285714 0.15714286 0.17142857 0.18571429 0.2 0.21428571 0.22857143 0.24285714 0.25714286 0.27142857 0.28571429 0.3 0.31428571 0.32857143 0.34285714 0.35714286 0.37142857 0.38571429 0.4 0.41428571 0.42857143 0.44285714 0.45714286 0.47142857 0.48571429 0.5 0.51428571 0.52857143 0.54285714 0.55714286 0.57142857 0.58571429 0.6 0.61428571 0.62857143 0.64285714 0.65714286 0.67142857 0.68571429 0.7 0.71428571 0.72857143 0.74285714 0.75714286 0.77142857 0.78571429 0.8 0.81428571 0.82857143 0.84285714 0.85714286 0.87142857 0.88571429 0.9 0.91428571 0.92857143 0.94285714 0.95714286 0.97142857 0.98571429 1 1 1 1 1 1
  arc A134 (3.3339, -26.4547) -> (3.714, -26.3528) centre (1.6741, -19.5) ccw
  spline S63 degree 5 poles (3.714, -26.3528) (3.7148, -26.3498) (3.7162, -26.3438) (3.7183, -26.3348) (3.721, -26.3228) (3.7244, -26.3078) (3.7277, -26.2928) (3.7309, -26.2778) (3.734, -26.2628) (3.7371, -26.2478) (3.7401, -26.2329) (3.743, -26.2179) (3.7459, -26.203) (3.7487, -26.1881) (3.7514, -26.1731) (3.754, -26.1582) (3.7566, -26.1433) (3.7591, -26.1285) (3.7615, -26.1136) (3.7638, -26.0987) (3.7661, -26.0839) (3.7683, -26.0691) (3.7704, -26.0542) (3.7724, -26.0394) (3.7743, -26.0247) (3.7762, -26.0099) (3.778, -25.9951) (3.7797, -25.9804) (3.7813, -25.9656) (3.7829, -25.9509) (3.7844, -25.9362) (3.7857, -25.9216) (3.787, -25.9069) (3.7883, -25.8923) (3.7894, -25.8776) (3.7905, -25.863) (3.7914, -25.8484) (3.7923, -25.8339) (3.7931, -25.8193) (3.7938, -25.8048) (3.7944, -25.7903) (3.7949, -25.7758) (3.7954, -25.7613) (3.7957, -25.7469) (3.796, -25.7325) (3.7961, -25.7181) (3.7962, -25.7037) (3.7962, -25.6894) (3.796, -25.675) (3.7958, -25.6607) (3.7955, -25.6465) (3.795, -25.6322) (3.7945, -25.618) (3.7938, -25.6039) (3.793, -25.5897) (3.7921, -25.5756) (3.7912, -25.5615) (3.7901, -25.5475) (3.7889, -25.5334) (3.7876, -25.5194) (3.7861, -25.5055) (3.7845, -25.4916) (3.7827, -25.4778) (3.7807, -25.464) (3.7786, -25.4502) (3.7763, -25.4365) (3.774, -25.4229) (3.7716, -25.4092) (3.769, -25.3956) (3.7662, -25.3821) (3.7631, -25.3687) (3.7601, -25.3581) (3.7577, -25.3503) (3.7559, -25.3451) (3.755, -25.3425) knots -1 -1 -1 -1 -1 -1 -0.98571429 -0.97142857 -0.95714286 -0.94285714 -0.92857143 -0.91428571 -0.9 -0.88571429 -0.87142857 -0.85714286 -0.84285714 -0.82857143 -0.81428571 -0.8 -0.78571429 -0.77142857 -0.75714286 -0.74285714 -0.72857143 -0.71428571 -0.7 -0.68571429 -0.67142857 -0.65714286 -0.64285714 -0.62857143 -0.61428571 -0.6 -0.58571429 -0.57142857 -0.55714286 -0.54285714 -0.52857143 -0.51428571 -0.5 -0.48571429 -0.47142857 -0.45714286 -0.44285714 -0.42857143 -0.41428571 -0.4 -0.38571429 -0.37142857 -0.35714286 -0.34285714 -0.32857143 -0.31428571 -0.3 -0.28571429 -0.27142857 -0.25714286 -0.24285714 -0.22857143 -0.21428571 -0.2 -0.18571429 -0.17142857 -0.15714286 -0.14285714 -0.12857143 -0.11428571 -0.1 -0.08571429 -0.07142857 -0.05714286 -0.04285714 -0.02857143 -0.01428571 0 0 0 0 0 0
  line L71 (3.755, -25.3425) -> (3.7322, -25.2779)
  arc A135 (3.8745, -24.9627) -> (3.7322, -25.2779) centre (3.9679, -25.1946) ccw
  arc A136 (3.8745, -24.9627) -> (3.981, -24.9186) centre (1.6741, -19.5) ccw
  arc A137 (4.3045, -25.0408) -> (3.981, -24.9186) centre (4.0789, -25.1486) ccw
  line L72 (4.3045, -25.0408) -> (4.334, -25.1026)
  spline S64 degree 5 poles (4.334, -25.1026) (4.3352, -25.1051) (4.3376, -25.1101) (4.3414, -25.1174) (4.3469, -25.1269) (4.3541, -25.1386) (4.3617, -25.1501) (4.3695, -25.1616) (4.3774, -25.1729) (4.3854, -25.1842) (4.3935, -25.1955) (4.4017, -25.2067) (4.4101, -25.2179) (4.4186, -25.2289) (4.4273, -25.2399) (4.4361, -25.2508) (4.4451, -25.2616) (4.4541, -25.2724) (4.4633, -25.2831) (4.4726, -25.2937) (4.4819, -25.3044) (4.4914, -25.3149) (4.5009, -25.3254) (4.5106, -25.3358) (4.5204, -25.3462) (4.5302, -25.3565) (4.5402, -25.3668) (4.5502, -25.377) (4.5603, -25.3872) (4.5705, -25.3973) (4.5808, -25.4074) (4.5912, -25.4174) (4.6016, -25.4274) (4.6122, -25.4373) (4.6228, -25.4472) (4.6335, -25.457) (4.6442, -25.4668) (4.6551, -25.4765) (4.666, -25.4862) (4.677, -25.4958) (4.6881, -25.5054) (4.6992, -25.5149) (4.7104, -25.5244) (4.7217, -25.5339) (4.7331, -25.5433) (4.7445, -25.5526) (4.756, -25.5619) (4.7676, -25.5712) (4.7792, -25.5804) (4.7909, -25.5896) (4.8027, -25.5987) (4.8145, -25.6078) (4.8264, -25.6168) (4.8384, -25.6258) (4.8504, -25.6347) (4.8625, -25.6436) (4.8747, -25.6525) (4.8869, -25.6613) (4.8992, -25.6701) (4.9115, -25.6788) (4.9239, -25.6875) (4.9364, -25.6961) (4.9489, -25.7047) (4.9615, -25.7132) (4.9741, -25.7217) (4.9868, -25.7302) (4.9996, -25.7386) (5.0124, -25.747) (5.0253, -25.7553) (5.0382, -25.7636) (5.0512, -25.7718) (5.0617, -25.7783) (5.0695, -25.7832) (5.0748, -25.7865) (5.0774, -25.7881) knots 0 0 0 0 0 0 0.01428571 0.02857143 0.04285714 0.05714286 0.07142857 0.08571429 0.1 0.11428571 0.12857143 0.14285714 0.15714286 0.17142857 0.18571429 0.2 0.21428571 0.22857143 0.24285714 0.25714286 0.27142857 0.28571429 0.3 0.31428571 0.32857143 0.34285714 0.35714286 0.37142857 0.38571429 0.4 0.41428571 0.42857143 0.44285714 0.45714286 0.47142857 0.48571429 0.5 0.51428571 0.52857143 0.54285714 0.55714286 0.57142857 0.58571429 0.6 0.61428571 0.62857143 0.64285714 0.65714286 0.67142857 0.68571429 0.7 0.71428571 0.72857143 0.74285714 0.75714286 0.77142857 0.78571429 0.8 0.81428571 0.82857143 0.84285714 0.85714286 0.87142857 0.88571429 0.9 0.91428571 0.92857143 0.94285714 0.95714286 0.97142857 0.98571429 1 1 1 1 1 1
  arc A138 (5.0774, -25.7881) -> (5.4182, -25.5914) centre (1.6741, -19.5) ccw
  spline S65 degree 5 poles (5.4182, -25.5914) (5.4181, -25.5883) (5.4179, -25.5821) (5.4176, -25.5729) (5.4171, -25.5605) (5.4165, -25.5452) (5.4158, -25.5298) (5.415, -25.5145) (5.4142, -25.4992) (5.4133, -25.484) (5.4123, -25.4688) (5.4113, -25.4536) (5.4102, -25.4384) (5.409, -25.4232) (5.4078, -25.4081) (5.4064, -25.3931) (5.4051, -25.378) (5.4036, -25.363) (5.4021, -25.348) (5.4005, -25.333) (5.3988, -25.3181) (5.3971, -25.3032) (5.3953, -25.2884) (5.3934, -25.2735) (5.3915, -25.2588) (5.3895, -25.244) (5.3874, -25.2293) (5.3852, -25.2146) (5.383, -25.2) (5.3807, -25.1853) (5.3783, -25.1708) (5.3758, -25.1562) (5.3733, -25.1417) (5.3707, -25.1273) (5.368, -25.1128) (5.3652, -25.0985) (5.3624, -25.0841) (5.3595, -25.0698) (5.3565, -25.0556) (5.3534, -25.0413) (5.3502, -25.0272) (5.347, -25.013) (5.3437, -24.999) (5.3402, -24.9849) (5.3368, -24.9709) (5.3332, -24.957) (5.3295, -24.9431) (5.3258, -24.9292) (5.3219, -24.9154) (5.318, -24.9017) (5.314, -24.888) (5.3099, -24.8744) (5.3057, -24.8608) (5.3014, -24.8473) (5.297, -24.8338) (5.2924, -24.8204) (5.2879, -24.807) (5.2832, -24.7937) (5.2784, -24.7805) (5.2735, -24.7673) (5.2685, -24.7542) (5.2633, -24.7412) (5.258, -24.7283) (5.2525, -24.7155) (5.2469, -24.7028) (5.2412, -24.6902) (5.2354, -24.6776) (5.2295, -24.665) (5.2235, -24.6525) (5.2173, -24.6402) (5.2108, -24.6281) (5.2053, -24.6186) (5.2009, -24.6117) (5.1978, -24.6071) (5.1962, -24.6048) knots -1 -1 -1 -1 -1 -1 -0.98571429 -0.97142857 -0.95714286 -0.94285714 -0.92857143 -0.91428571 -0.9 -0.88571429 -0.87142857 -0.85714286 -0.84285714 -0.82857143 -0.81428571 -0.8 -0.78571429 -0.77142857 -0.75714286 -0.74285714 -0.72857143 -0.71428571 -0.7 -0.68571429 -0.67142857 -0.65714286 -0.64285714 -0.62857143 -0.61428571 -0.6 -0.58571429 -0.57142857 -0.55714286 -0.54285714 -0.52857143 -0.51428571 -0.5 -0.48571429 -0.47142857 -0.45714286 -0.44285714 -0.42857143 -0.41428571 -0.4 -0.38571429 -0.37142857 -0.35714286 -0.34285714 -0.32857143 -0.31428571 -0.3 -0.28571429 -0.27142857 -0.25714286 -0.24285714 -0.22857143 -0.21428571 -0.2 -0.18571429 -0.17142857 -0.15714286 -0.14285714 -0.12857143 -0.11428571 -0.1 -0.08571429 -0.07142857 -0.05714286 -0.04285714 -0.02857143 -0.01428571 0 0 0 0 0 0
  line L73 (5.1962, -24.6048) -> (5.1575, -24.5484)
  arc A139 (5.2134, -24.2071) -> (5.1575, -24.5484) centre (5.3636, -24.4069) ccw
  arc A140 (5.2134, -24.2071) -> (5.3048, -24.1369) centre (1.6741, -19.5) ccw
  arc A141 (5.6489, -24.1713) -> (5.3048, -24.1369) centre (5.4589, -24.3338) ccw
  line L74 (5.6489, -24.1713) -> (5.6934, -24.2233)
  spline S66 degree 5 poles (5.6934, -24.2233) (5.6952, -24.2254) (5.6988, -24.2295) (5.7044, -24.2356) (5.7121, -24.2434) (5.7222, -24.2529) (5.7325, -24.262) (5.743, -24.271) (5.7536, -24.2799) (5.7642, -24.2888) (5.775, -24.2976) (5.7858, -24.3063) (5.7968, -24.3149) (5.8078, -24.3234) (5.8191, -24.3318) (5.8304, -24.34) (5.8419, -24.3481) (5.8534, -24.3562) (5.8651, -24.3641) (5.8768, -24.372) (5.8885, -24.3799) (5.9004, -24.3876) (5.9123, -24.3953) (5.9244, -24.4029) (5.9365, -24.4104) (5.9487, -24.4178) (5.9609, -24.4251) (5.9733, -24.4324) (5.9857, -24.4396) (5.9982, -24.4467) (6.0107, -24.4538) (6.0233, -24.4608) (6.036, -24.4677) (6.0487, -24.4746) (6.0615, -24.4814) (6.0744, -24.4881) (6.0873, -24.4947) (6.1003, -24.5013) (6.1134, -24.5078) (6.1265, -24.5143) (6.1397, -24.5207) (6.1529, -24.527) (6.1662, -24.5333) (6.1796, -24.5395) (6.193, -24.5456) (6.2064, -24.5517) (6.22, -24.5577) (6.2335, -24.5637) (6.2471, -24.5696) (6.2608, -24.5754) (6.2746, -24.5812) (6.2883, -24.5869) (6.3022, -24.5925) (6.3161, -24.5981) (6.33, -24.6036) (6.344, -24.6091) (6.358, -24.6145) (6.3721, -24.6198) (6.3862, -24.6251) (6.4004, -24.6304) (6.4146, -24.6355) (6.4289, -24.6406) (6.4432, -24.6457) (6.4576, -24.6507) (6.472, -24.6556) (6.4865, -24.6605) (6.501, -24.6653) (6.5155, -24.6701) (6.5301, -24.6748) (6.5447, -24.6794) (6.5594, -24.684) (6.5712, -24.6877) (6.58, -24.6904) (6.586, -24.6921) (6.5889, -24.693) knots 0 0 0 0 0 0 0.01428571 0.02857143 0.04285714 0.05714286 0.07142857 0.08571429 0.1 0.11428571 0.12857143 0.14285714 0.15714286 0.17142857 0.18571429 0.2 0.21428571 0.22857143 0.24285714 0.25714286 0.27142857 0.28571429 0.3 0.31428571 0.32857143 0.34285714 0.35714286 0.37142857 0.38571429 0.4 0.41428571 0.42857143 0.44285714 0.45714286 0.47142857 0.48571429 0.5 0.51428571 0.52857143 0.54285714 0.55714286 0.57142857 0.58571429 0.6 0.61428571 0.62857143 0.64285714 0.65714286 0.67142857 0.68571429 0.7 0.71428571 0.72857143 0.74285714 0.75714286 0.77142857 0.78571429 0.8 0.81428571 0.82857143 0.84285714 0.85714286 0.87142857 0.88571429 0.9 0.91428571 0.92857143 0.94285714 0.95714286 0.97142857 0.98571429 1 1 1 1 1 1
  arc A142 (6.5889, -24.693) -> (6.8672, -24.4148) centre (1.6741, -19.5) ccw
  spline S67 degree 5 poles (6.8672, -24.4148) (6.8663, -24.4118) (6.8645, -24.4059) (6.8618, -24.3971) (6.8582, -24.3853) (6.8536, -24.3706) (6.8489, -24.356) (6.8442, -24.3414) (6.8395, -24.3268) (6.8346, -24.3123) (6.8298, -24.2979) (6.8248, -24.2834) (6.8198, -24.2691) (6.8148, -24.2548) (6.8097, -24.2405) (6.8045, -24.2263) (6.7993, -24.2121) (6.794, -24.198) (6.7886, -24.1839) (6.7832, -24.1698) (6.7778, -24.1558) (6.7722, -24.1419) (6.7666, -24.128) (6.761, -24.1142) (6.7553, -24.1004) (6.7495, -24.0867) (6.7437, -24.073) (6.7378, -24.0594) (6.7319, -24.0458) (6.7258, -24.0323) (6.7198, -24.0188) (6.7136, -24.0054) (6.7074, -23.9921) (6.7012, -23.9788) (6.6948, -23.9656) (6.6884, -23.9524) (6.682, -23.9393) (6.6755, -23.9262) (6.6689, -23.9132) (6.6622, -23.9003) (6.6555, -23.8874) (6.6487, -23.8746) (6.6419, -23.8619) (6.6349, -23.8492) (6.6279, -23.8366) (6.6209, -23.824) (6.6137, -23.8115) (6.6065, -23.7991) (6.5993, -23.7868) (6.5919, -23.7745) (6.5845, -23.7623) (6.577, -23.7502) (6.5694, -23.7382) (6.5617, -23.7263) (6.554, -23.7144) (6.5462, -23.7026) (6.5383, -23.6909) (6.5303, -23.6793) (6.5223, -23.6677) (6.5141, -23.6563) (6.5059, -23.6449) (6.4975, -23.6337) (6.4891, -23.6226) (6.4805, -23.6117) (6.4717, -23.6008) (6.4629, -23.5901) (6.4541, -23.5794) (6.4452, -23.5688) (6.4362, -23.5583) (6.427, -23.548) (6.4176, -23.538) (6.4097, -23.5303) (6.4037, -23.5247) (6.3995, -23.5211) (6.3975, -23.5193) knots -1 -1 -1 -1 -1 -1 -0.98571429 -0.97142857 -0.95714286 -0.94285714 -0.92857143 -0.91428571 -0.9 -0.88571429 -0.87142857 -0.85714286 -0.84285714 -0.82857143 -0.81428571 -0.8 -0.78571429 -0.77142857 -0.75714286 -0.74285714 -0.72857143 -0.71428571 -0.7 -0.68571429 -0.67142857 -0.65714286 -0.64285714 -0.62857143 -0.61428571 -0.6 -0.58571429 -0.57142857 -0.55714286 -0.54285714 -0.52857143 -0.51428571 -0.5 -0.48571429 -0.47142857 -0.45714286 -0.44285714 -0.42857143 -0.41428571 -0.4 -0.38571429 -0.37142857 -0.35714286 -0.34285714 -0.32857143 -0.31428571 -0.3 -0.28571429 -0.27142857 -0.25714286 -0.24285714 -0.22857143 -0.21428571 -0.2 -0.18571429 -0.17142857 -0.15714286 -0.14285714 -0.12857143 -0.11428571 -0.1 -0.08571429 -0.07142857 -0.05714286 -0.04285714 -0.02857143 -0.01428571 0 0 0 0 0 0
  line L75 (6.3975, -23.5193) -> (6.3454, -23.4748)
  arc A143 (6.3111, -23.1307) -> (6.3454, -23.4748) centre (6.5079, -23.2848) ccw
  arc A144 (6.3111, -23.1307) -> (6.3812, -23.0392) centre (1.6741, -19.5) ccw
  arc A145 (6.7225, -22.9833) -> (6.3812, -23.0392) centre (6.581, -23.1895) ccw
  line L76 (6.7225, -22.9833) -> (6.779, -23.0221)
  spline S68 degree 5 poles (6.779, -23.0221) (6.7812, -23.0237) (6.7858, -23.0267) (6.7928, -23.0311) (6.8022, -23.0367) (6.8144, -23.0432) (6.8267, -23.0494) (6.8391, -23.0554) (6.8517, -23.0612) (6.8643, -23.067) (6.877, -23.0728) (6.8897, -23.0784) (6.9025, -23.0838) (6.9154, -23.0892) (6.9284, -23.0943) (6.9415, -23.0994) (6.9546, -23.1043) (6.9679, -23.109) (6.9812, -23.1137) (6.9945, -23.1183) (7.0079, -23.1228) (7.0214, -23.1272) (7.0349, -23.1315) (7.0485, -23.1358) (7.0621, -23.1399) (7.0758, -23.1439) (7.0896, -23.1478) (7.1034, -23.1516) (7.1172, -23.1554) (7.1311, -23.159) (7.1451, -23.1626) (7.1591, -23.1661) (7.1731, -23.1695) (7.1872, -23.1728) (7.2013, -23.1761) (7.2155, -23.1792) (7.2297, -23.1823) (7.244, -23.1853) (7.2583, -23.1882) (7.2726, -23.1911) (7.287, -23.1938) (7.3014, -23.1965) (7.3159, -23.1991) (7.3304, -23.2017) (7.3449, -23.2041) (7.3595, -23.2065) (7.3741, -23.2088) (7.3887, -23.2111) (7.4034, -23.2132) (7.4181, -23.2153) (7.4329, -23.2173) (7.4477, -23.2193) (7.4625, -23.2212) (7.4774, -23.223) (7.4923, -23.2247) (7.5072, -23.2264) (7.5221, -23.228) (7.5371, -23.2295) (7.5521, -23.2309) (7.5672, -23.2323) (7.5823, -23.2336) (7.5974, -23.2349) (7.6125, -23.236) (7.6277, -23.2371) (7.6429, -23.2382) (7.6581, -23.2391) (7.6734, -23.24) (7.6887, -23.2409) (7.704, -23.2417) (7.7193, -23.2424) (7.7347, -23.243) (7.747, -23.2434) (7.7562, -23.2438) (7.7624, -23.2439) (7.7655, -23.244) knots 0 0 0 0 0 0 0.01428571 0.02857143 0.04285714 0.05714286 0.07142857 0.08571429 0.1 0.11428571 0.12857143 0.14285714 0.15714286 0.17142857 0.18571429 0.2 0.21428571 0.22857143 0.24285714 0.25714286 0.27142857 0.28571429 0.3 0.31428571 0.32857143 0.34285714 0.35714286 0.37142857 0.38571429 0.4 0.41428571 0.42857143 0.44285714 0.45714286 0.47142857 0.48571429 0.5 0.51428571 0.52857143 0.54285714 0.55714286 0.57142857 0.58571429 0.6 0.61428571 0.62857143 0.64285714 0.65714286 0.67142857 0.68571429 0.7 0.71428571 0.72857143 0.74285714 0.75714286 0.77142857 0.78571429 0.8 0.81428571 0.82857143 0.84285714 0.85714286 0.87142857 0.88571429 0.9 0.91428571 0.92857143 0.94285714 0.95714286 0.97142857 0.98571429 1 1 1 1 1 1
  arc A146 (7.7655, -23.244) -> (7.9623, -22.9033) centre (1.6741, -19.5) ccw